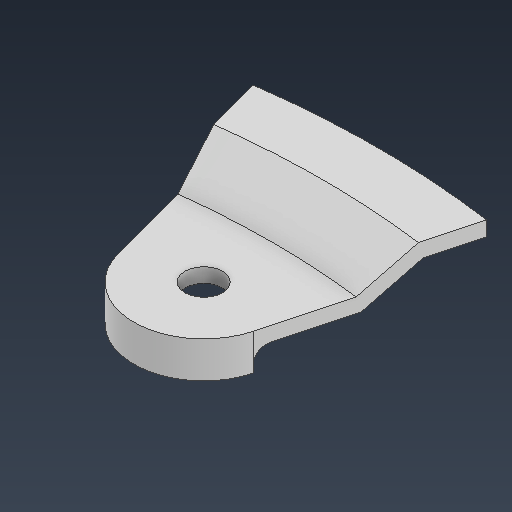
# Autodesk Inventor part: transmission_support
Saved by Autodesk Inventor 2025.3 (Build 293356000, 356)
## iProperties
Created: 2025-11-28
Part Number: transmission_support
Material: 一般
Document SubType Name: Modeling
Designer: 陳泓任
Density: 1 g/cm^3
Appearance: 預設
Author: 陳泓任
Autodesk Inventor part; units mm, degrees
ref_plane "YZ Plane" through (0, 0, 0) normal (1, 0, 0) x (0, 1, 0)
ref_plane "XZ Plane" through (0, 0, 0) normal (0, 1, 0) x (-1, 0, 0)
ref_plane "XY Plane" through (0, 0, 0) normal (0, 0, 1) x (1, 0, 0)
sketch "草圖5" plane through (0, 0, 0) normal (0, 0, 1) x (1, 0, 0)
  line L0 (0, 14.1091) -> (0, -11.8545)
  line L1 (-92, 0) -> (-102, 0)
  line L2 (-102, 0) -> (-108.9282, 4)
  line L3 (-108.9282, 4) -> (-116, 4)
  line L4 (-116, 4) -> (-116, 6)
  line L5 (-116, 6) -> (-108.3923, 6)
  line L6 (-108.3923, 6) -> (-101.4641, 2)
  line L7 (-101.4641, 2) -> (-92, 2)
  line L8 (-92, 4.8545) -> (-92, -2.1478) construction
  line L9 (-92, 0) -> (-82, 0)
  line L10 (-82, 0) -> (-82, 2)
  line L11 (-82, 2) -> (-92, 2)
  point P0 (0, 0)
  point P1 (0, 2)
  dimension "d26" = 2
  dimension "d27" = 232
  dimension "d28" = 92
  dimension "d31" = 2
  dimension "d32" = 2
  dimension "d33" = 4
  dimension "d34" = 30
  dimension "d35" = 20
  constraints: 24 end point, 5 perpendicular, 5 point on line, 2 horizontal, 2 vertical, 1 parallel, 1 symmetric about line
  measures "d26" distance of L3.end L4.end
  measures "d27" diameter of L4 L0
  measures "d28" distance between parallel lines of L8 L0
  measures "d31" distance between parallel lines of L1 L7
  measures "d32" distance between parallel lines of L2 L6
  measures "d33" distance between parallel lines of L1 L3
  measures "d34" angle of L1 L2
  measures "d35" diameter of L1.end L8
revolve "迴轉1" add sketch "草圖5" angle 360 about axis through (0, 14.1091, 0) along (0, -1, 0)
sketch "草圖6" plane through (0, 0, 0) normal (0, 1, 0) x (-1, 0, 0)
  circle A0 centre (0, -92) radius 2.58
  line L0 (0, -136.9187) -> (0, 28.2306) construction
  line L1 (-16.0697, -114.8815) -> (-9.2729, -89.5153)
  arc A1 (7.341, -90.033) -> (-7.341, -90.033) centre (0, -92) ccw
  line L2 (16.0697, -114.8815) -> (9.2729, -89.5153)
  arc A2 (-16.0697, -114.8815) -> (16.0697, -114.8815) centre (0, 0) ccw
  circle A3 centre (0, 0) radius 116 construction
  arc A4 (9.2729, -89.5153) -> (-9.2729, -89.5153) centre (0, -92) ccw
  arc A5 (-9.7984, -91.4767) -> (9.7984, -91.4767) centre (0, 0) ccw construction
  line L3 (-7.341, -90.033) -> (-9.2729, -89.5153)
  line L4 (7.341, -90.033) -> (9.2729, -89.5153)
  arc A6 (7.2444, -90.0589) -> (-7.2207, -89.9724) centre (0, -92) ccw construction
  point P0 (-9.2729, -89.5153)
  dimension "d38" = 92
  dimension "d46" = 5.16
  dimension "d81" = 7.6
  dimension "d82" = 2
  dimension "d83" = 30
  dimension "d88" = 7.5
  constraints: 11 point on circle, 10 end point, 6 centre point, 5 coincident, 5 point on line, 2 concentric, 2 tangent, 1 line through centre, 1 symmetric about line, 1 vertical, 2 other
  measures "d38" distance of point (0, 0) A0.centre
  measures "d46" diameter of A0
  measures "d81" radius of A1
  measures "d82" radial gap between concentric circles of A4 A1
  measures "d83" angle of L2 L1
  measures "d88" radius of A6
extrude "擠出5" cut sketch "草圖6" along normal up to next contours A0
extrude "擠出8" cut sketch "草圖6" along normal blind 10 keep common part
extrude "擠出9" add sketch "草圖6" against normal blind 3 contours A4 L4 A1 L3
fillet "圓角5" radius 2 2 edges at (8.307, 0, -89.7742) (-8.307, 0, -89.7742)
